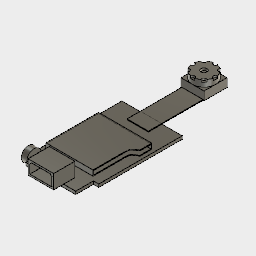
3202 Spy Camera (Autodesk Fusion 360 design; units mm, degrees)
Autodesk Fusion 360 part; units mm, degrees
sketch "pcb" plane through (0, 0, 0) normal (0, 0, 1) x (1, 0, 0)
  line L0 (0, 0) -> (17, 0)
  line L1 (17, 0) -> (17, 28.5)
  line L2 (17, 28.5) -> (0, 28.5)
  line L3 (0, 28.5) -> (0, 0)
  line L4 (1, 6.1) -> (16, 6.1)
  line L5 (16, 6.1) -> (16, 20.9)
  line L6 (16, 20.9) -> (1, 20.9)
  line L7 (1, 20.9) -> (1, 6.1)
  line L8 (8.5, 0) -> (8.5, 28.5) construction
  line L9 (8.5, 6.1) -> (8.5, 20.9) construction
  line L10 (14.2667, 6.1) -> (14.2667, 15)
  spline S0 degree 2 poles (14.2667, 15) (14.3, 16.5) (16, 17.5579) knots 0 0 0 0.332603 0.332603 0.332603 weights 1 3 1
  line L11 (1.5, 0) -> (1.5, 5)
  line L12 (1.5, 5) -> (0, 5)
  line L13 (15.5, 0) -> (15.5, 5)
  line L14 (15.5, 5) -> (17, 5)
  dimension "d1" = 17
  dimension "d2" = 28.5
  dimension "d3" = 15
  dimension "d4" = 14.8
  dimension "d5" = 7.6
  dimension "d10" = 5
  dimension "d11" = 1.5
  measures "d1" distance of L0.start L0.end
  measures "d2" distance of L0.start L2.end
  measures "d3" distance of L4.start L4.end
  measures "d4" distance of L4.start L6.end
  measures "d5" distance of L2 L6
  measures "d10" distance of L11.start L11.end
  measures "d11" distance of L11.end L12.end
extrude "Extrude1" add sketch "pcb" against normal blind 0.85 contours L0 L1 L2 L3 L11 L12 L13 L14 | L4 L5 L6 L7 L10 S0 | L4 L5 L10 S0 makes body 1
extrude "Extrude2" add sketch "pcb" along normal blind 1.5 separate body contours L4 L5 L6 L7 L10 S0 makes body 2
sketch "usb" plane through (0, 0, 0) normal (0, 0, 1) x (-1, 0, 0)
  line L0 (-1.5, 0) -> (-15.5, 0)
  line L1 (-15.5, 0) -> (-15.5, -5)
  line L2 (-15.5, -5) -> (-17, -5)
  line L3 (-17, -5) -> (-17, -28.5)
  line L4 (-17, -28.5) -> (0, -28.5)
  line L5 (0, -28.5) -> (0, -5)
  line L6 (0, -5) -> (-1.5, -5)
  line L7 (-1.5, -5) -> (-1.5, 0)
  line L8 (-8.5, 0) -> (-8.5, -28.5) construction
  line L9 (-4.9, 2.8) -> (-12.1, 2.8)
  line L10 (-12.1, 2.8) -> (-12.1, -3.2)
  line L11 (-12.1, -3.2) -> (-4.9, -3.2)
  line L12 (-4.9, -3.2) -> (-4.9, 2.8)
  line L13 (-8.5, 2.8) -> (-8.5, -3.2) construction
  dimension "d12" = 7.2
  dimension "d13" = 6
  dimension "d14" = 2.8
  measures "d12" distance of L9.start L9.end
  measures "d13" distance of L9.start L11.end
  measures "d14" distance of L0 L9
extrude "Extrude3" add sketch "usb" along normal blind 4 separate body contours L0 L10 L11 L12 | L0 L9 L10 L12 makes body 3
sketch "mic" plane through (1.5, 0, 0) normal (-1, 0, 0) x (0, -1, 0)
  line L0 (0, 0) -> (-5, 0)
  line L1 (-5, 0) -> (-5, -0.85)
  line L2 (-5, -0.85) -> (0, -0.85)
  line L3 (0, -0.85) -> (0, 0)
  circle A0 centre (-2.5, 0) radius 2
  dimension "d17" = 4
  measures "d17" diameter of A0
extrude "Extrude4" add sketch "mic" along normal blind 1.8 and the other way blind -0.2 separate body contours L0 L2 A0 | L0 A0 | L2 A0 makes body 4
shell "Shell1" thickness 0.2 removed faces 3 at (14.2667, 9.0667, 1) at (16, 18.6719, 0.5) at (15.7818, 17.4214, 0.75) on bodies 2
shell "Shell2" thickness 0.5 removed faces 1 at (7.3, -2.8, 1.3333) on bodies 3
chamfer "Chamfer1" distance 0.5 angle 45 2 edges at (5.4, -0.05, 3.5) (11.6, -0.05, 3.5) on bodies 3
sketch "chips" plane through (0, 0, -0.85) normal (0, 0, -1) x (1, 0, 0)
  line L0 (15.5, 0) -> (1.5, 0)
  line L1 (1.5, 0) -> (1.5, -5)
  line L2 (1.5, -5) -> (0, -5)
  line L3 (0, -5) -> (0, -28.5)
  line L4 (0, -28.5) -> (17, -28.5)
  line L5 (17, -28.5) -> (17, -5)
  line L6 (17, -5) -> (15.5, -5)
  line L7 (15.5, -5) -> (15.5, 0)
  line L8 (4, -15.5) -> (11, -15.5)
  line L9 (11, -15.5) -> (11, -8.5)
  line L10 (11, -8.5) -> (4, -8.5)
  line L11 (4, -8.5) -> (4, -15.5)
  line L12 (4, -15.5) -> (11, -8.5) construction
  line L13 (11, -15.5) -> (4, -8.5) construction
  line L14 (9.8, -26.7) -> (13.6, -26.7)
  line L15 (13.6, -26.7) -> (13.6, -21.7)
  line L16 (13.6, -21.7) -> (9.8, -21.7)
  line L17 (9.8, -21.7) -> (9.8, -26.7)
  line L18 (9.8, -26.7) -> (13.6, -21.7) construction
  line L19 (13.6, -26.7) -> (9.8, -21.7) construction
  point P0 (7.5, -12)
  point P1 (11.7, -24.2)
  dimension "d25" = 7
  dimension "d26" = 7
  dimension "d27" = 4
  dimension "d28" = 8.5
  dimension "d29" = 3.8
  dimension "d30" = 5
  dimension "d31" = 3.4
  dimension "d32" = 1.8
  measures "d25" distance of L9.end L10.end
  measures "d26" distance of L8.end L9.end
  measures "d27" distance of L3 L11
  measures "d28" distance of L0 L10
  measures "d29" distance of L15.end L16.end
  measures "d30" distance of L14.end L15.end
  measures "d31" distance of L5 L15
  measures "d32" distance of L4 L14
extrude "Extrude5" add sketch "chips" along normal blind 1.6 contours L8 L9 L10 L11 | L14 L15 L16 L17 bodies 1
sketch "cam" plane through (0, 0, 0) normal (0, 0, 1) x (-1, 0, 0)
  line L0 (-1.5, 0) -> (-15.5, 0)
  line L1 (-15.5, 0) -> (-15.5, -5)
  line L2 (-15.5, -5) -> (-17, -5)
  line L3 (-17, -5) -> (-17, -28.5)
  line L4 (-17, -28.5) -> (0, -28.5)
  line L5 (0, -28.5) -> (0, -5)
  line L6 (0, -5) -> (-1.5, -5)
  line L7 (-1.5, -5) -> (-1.5, 0)
  line L8 (-5, -25) -> (-11, -25)
  line L9 (-11, -25) -> (-11, -40.4)
  line L10 (-11, -40.4) -> (-5, -40.4)
  line L11 (-5, -40.4) -> (-5, -25)
  line L12 (-8, -40.4) -> (-8, -25) construction
  line L13 (-11.25, -40.4) -> (-4.75, -40.4)
  line L14 (-4.75, -40.4) -> (-4.75, -46.9)
  line L15 (-4.75, -46.9) -> (-11.25, -46.9)
  line L16 (-11.25, -46.9) -> (-11.25, -40.4)
  line L17 (-11.25, -40.4) -> (-4.75, -46.9) construction
  line L18 (-4.75, -40.4) -> (-11.25, -46.9) construction
  point P0 (-8, -43.65)
  dimension "d35" = 6
  dimension "d36" = 15.4
  dimension "d37" = 3.5
  dimension "d38" = 6.5
  dimension "d39" = 6.5
  measures "d35" distance of L8.start L8.end
  measures "d36" distance of L8.start L10.end
  measures "d37" distance of L4 L8
  measures "d38" distance of L14.end L15.end
  measures "d39" distance of L13.end L14.end
extrude "Extrude6" add sketch "cam" along normal blind 0.2 separate body contours L4 L9 L10 L11 L13 | L4 L8 L9 L11 makes body 5
extrude "Extrude7" add sketch "cam" along normal blind 2.4 contours L10 L13 L14 L15 L16 bodies 5
sketch "iris" plane through (0, 0, 2.4) normal (0, 0, 1) x (-1, 0, 0)
  line L0 (-11.25, -46.9) -> (-4.75, -46.9)
  line L1 (-4.75, -46.9) -> (-4.75, -40.4)
  line L2 (-4.75, -40.4) -> (-11.25, -40.4)
  line L3 (-11.25, -40.4) -> (-11.25, -46.9)
  circle A0 centre (-8, -43.65) radius 3.25
  point P0 (-8, -43.65)
extrude "Extrude8" add sketch "iris" along normal blind 1.8 contours A0 bodies 5 1
ref_plane "WorkPlane1" through (8.5, 13.5, -4.5) normal (0, 0, 1) x (1, 0, 0)
sketch "mount bot" plane through (8.5, 13.5, -4.5) normal (0, 0, 1) x (1, 0, 0)
  line L0 (-11, -17) -> (12, -17)
  line L1 (12, -17) -> (12, 17)
  line L2 (12, 17) -> (-11, 17)
  line L3 (-11, 17) -> (-11, -17)
extrude "Extrude9" add sketch "mount bot" along normal blind 1 separate body makes body 6
sketch "mount top" plane through (0, 0, -3.5) normal (0, 0, 1) x (-1, 0, 0)
  line L0 (2.5, -30.5) -> (2.5, 3.5)
  line L1 (2.5, 3.5) -> (-20.5, 3.5)
  line L2 (-20.5, 3.5) -> (-20.5, -30.5)
  line L3 (-20.5, -30.5) -> (2.5, -30.5)
  line L4 (-1.5, 0) -> (-15.5, 0) construction
  line L5 (-15.5, 0) -> (-15.5, -5) construction
  line L6 (-15.5, -5) -> (-17, -5) construction
  line L7 (-17, -5) -> (-17, -28.5) construction
  line L8 (-17, -28.5) -> (0, -28.5) construction
  line L9 (0, -28.5) -> (0, -5) construction
  line L10 (0, -5) -> (-1.5, -5) construction
  line L11 (-1.5, -5) -> (-1.5, 0) construction
  line L12 (2.5, -30.5) -> (-3, -30.5)
  line L13 (-3, -30.5) -> (-3, -25)
  line L14 (-3, -25) -> (2.5, -25)
  line L15 (2.5, -25) -> (2.5, -30.5)
  line L16 (-20.5, -30.5) -> (-15, -30.5)
  line L17 (-15, -30.5) -> (-15, -25)
  line L18 (-15, -25) -> (-20.5, -25)
  line L19 (-20.5, -25) -> (-20.5, -30.5)
  line L20 (-20.5, -4.8) -> (-15, -4.8)
  line L21 (-15, -4.8) -> (-15, -10.3)
  line L22 (-15, -10.3) -> (-20.5, -10.3)
  line L23 (-20.5, -10.3) -> (-20.5, -4.8)
  line L24 (2.5, -4.8) -> (-3, -4.8)
  line L25 (-3, -4.8) -> (-3, -10.3)
  line L26 (-3, -10.3) -> (2.5, -10.3)
  line L27 (2.5, -10.3) -> (2.5, -4.8)
  line L28 (-17, 2) -> (-12.5, 2)
  line L29 (-12.5, 2) -> (-12.5, -2.5)
  line L30 (-12.5, -2.5) -> (-17, -2.5)
  line L31 (-17, -2.5) -> (-17, 2)
  line L32 (-12.1, 2.8) -> (-12.1, -3.2)
  line L33 (-1.5, 2) -> (-4.5, 2)
  line L34 (-4.5, 2) -> (-4.5, -2)
  line L35 (-4.5, -2) -> (-1.5, -2)
  line L36 (-1.5, -2) -> (-1.5, 2)
  line L37 (-4.9, -3.2) -> (-4.9, 2.8)
  line L38 (-1.3, -4.8) -> (-1.3, 0.2)
  line L39 (-1.3, 0.2) -> (-15.7, 0.2)
  line L40 (-15.7, 0.2) -> (-15.7, -4.8)
  line L41 (-15.7, -4.8) -> (-17.2, -4.8)
  line L42 (-17.2, -4.8) -> (-17.2, -28.7)
  line L43 (-17.2, -28.7) -> (0.2, -28.7)
  line L44 (0.2, -28.7) -> (0.2, -4.8)
  line L45 (0.2, -4.8) -> (-1.3, -4.8)
  dimension "d49" = 0.2
  dimension "d50" = 5.5
  dimension "d51" = 5.5
  dimension "d52" = 5.5
  dimension "d53" = 5.5
  measures "d50" distance of L20.start L20.end
  measures "d51" distance of L20.start L22.end
  measures "d52" distance of L24.start L24.end
  measures "d53" distance of L24.start L26.end
extrude "Extrude10" add sketch "mount top" along normal blind 2.5 contours L13 L14 L43 L44 | L24 L25 L26 L44 L45 | L17 L18 L42 L43 | L20 L21 L22 L41 L42 bodies 6
extrude "Extrude11" add sketch "mount top" along normal blind 4 contours L0 L3 L12 L13 L14 L15 L43 L44 | L0 L24 L26 L27 L44 | L2 L3 L16 L17 L18 L19 L42 L43 | L2 L20 L22 L23 L42 bodies 6
extrude "Extrude12" add sketch "mount top" along normal blind 2.5 contours L33 L34 L36 L39 | L34 L35 L36 L39 | L29 L30 L39 L40 | L28 L29 L30 L31 L39 L40 bodies 6
extrude "Extrude13" add sketch "mount top" along normal blind 4 contours L33 L34 L36 L39 | L28 L29 L30 L31 L39 L40 bodies 6 3
sketch "Sketch9" plane through (0, 0, 4.2) normal (0, 0, 1) x (-1, 0, 0)
  circle A0 centre (-8, -43.65) radius 3.25
  circle A1 centre (-8, -43.65) radius 0.8382
  line L0 (-8, -43.65) -> (-8, -48.5) construction
  circle A2 centre (-8, -46.9) radius 0.6
  circle A3 centre (-5.7019, -45.9481) radius 0.6
  circle A4 centre (-4.75, -43.65) radius 0.6
  circle A5 centre (-5.7019, -41.3519) radius 0.6
  circle A6 centre (-8, -40.4) radius 0.6
  circle A7 centre (-10.2981, -41.3519) radius 0.6
  circle A8 centre (-11.25, -43.65) radius 0.6
  circle A9 centre (-10.2981, -45.9481) radius 0.6
  point P0 (-8, -46.9)
  dimension "d62" = 1.2
  dimension "d64" = 360
  measures "d62" diameter of A2
extrude "Extrude14" cut sketch "Sketch9" against normal blind 0.6 contours A0 A4 | A0 A5 | A0 A3 | A0 A6 | A0 A2 | A0 A7 | A0 A9 | A0 A8 picked at (-4.9434, -43.525) picked at (-5.8462, -41.4962) picked at (-5.8462, -45.8038) picked at (-8, -40.6041) picked at (-8, -46.6959) picked at (-10.163, -41.5049) picked at (-10.163, -45.7951) picked at (-11.0459, -43.65) bodies 5
extrude "Extrude15" cut sketch "Sketch9" against normal blind 0.5 draft -25 contours A1 bodies 5
move_body "MoveBody2" bodies 5 to x (1, 0, 0) y (0, 1, 0) z (0, 0, 1) at (0.3, -0.35, 0)
hidden bodies 6
named bodies: "PCB", "microSD", "usb", "mic", "cam", "mount"
